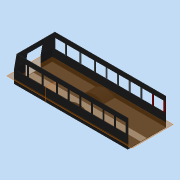
# Autodesk Inventor part: Pickle Interior
Saved by Autodesk Inventor 2018.2 (Build 222227000, 227)
## iProperties
Created: 2018-02-21
Part Number: Pickle Interior
Material: Generic
Document SubType Name: Modeling
Designer: owner
Density: 1 g/cm^3
Appearance: Default
Author: owner
Autodesk Inventor part; units mm, degrees
ref_plane "YZ Plane" through (0, 0, 0) normal (1, 0, 0) x (0, 1, 0)
ref_plane "XZ Plane" through (0, 0, 0) normal (0, 1, 0) x (-1, 0, 0)
ref_plane "XY Plane" through (0, 0, 0) normal (0, 0, 1) x (1, 0, 0)
sketch "Sketch1" plane through (0, 0, 0) normal (0, 1, 0) x (-1, 0, 0)
  line L0 (0, 0) -> (-6985, 0)
  line L1 (-6985, 0) -> (-6985, -2349.5)
  line L2 (-6985, -2349.5) -> (0, -2349.5)
  line L3 (0, -2349.5) -> (0, 0)
  dimension "d0" = 6985
  dimension "d1" = 2349.5
  constraints: 8 end point, 2 parallel, 1 horizontal, 1 perpendicular
  measures "d0" distance of L2.end L1.end
  measures "d1" distance of L1.end L0.end
extrude "Extrusion1" add sketch "Sketch1" along normal blind 25.4
sketch "Sketch2" plane through (0, 25.4, 0) normal (0, 1, 0) x (1, 0, 0)
  line L0 (0, 0) -> (6985, 0) projected
  line L1 (6985, 0) -> (6985, 2349.5) projected
  line L2 (6985, 2349.5) -> (0, 2349.5) projected
  line L3 (0, 2349.5) -> (0, 0) projected
  line L4 (6985, 25.4) -> (25.4, 25.4)
  line L5 (25.4, 25.4) -> (25.4, 2324.1)
  line L6 (25.4, 2324.1) -> (6985, 2324.1)
  dimension "d4" = 25.4
  constraints: 6 end point, 2 point on line
  measures "d4" distance between parallel lines of L0 L4
extrude "Extrusion2" add sketch "Sketch2" along normal blind 1644.65 contours L3 L2 L1 L6 L5 L4 L0
sketch "Sketch3" plane through (0, 0, 0) normal (0, 0, 1) x (1, 0, 0)
  line L0 (25.4, 25.4) -> (25.4, 742.95)
  line L1 (25.4, 742.95) -> (190.5, 742.95)
  line L2 (190.5, 742.95) -> (190.5, 1670.05)
  line L3 (25.4, 1670.05) -> (6985, 1670.05) projected
  line L4 (25.4, 742.95) -> (190.5, 1670.05)
  line L5 (190.5, 1670.05) -> (165.1, 1670.05)
  line L6 (165.1, 1670.05) -> (0, 742.95)
  line L7 (0, 0) -> (0, 1670.05) projected
  line L8 (0, 742.95) -> (0, 1670.05)
  line L9 (0, 1670.05) -> (165.1, 1670.05)
  line L10 (0, 742.95) -> (25.4, 742.95)
  dimension "d7" = 717.55
  dimension "d9" = 25.4
  constraints: 18 end point, 3 perpendicular, 3 point on line, 1 collinear, 1 parallel
  measures "d7" distance of L0.start L0.end
  measures "d9" distance of L2.end L5.end
extrude "Extrusion3" cut sketch "Sketch3" against normal up to surface (2349.5 mm away) contours L7 L9 L3 L6
extrude "Extrusion4" add sketch "Sketch3" against normal up to surface (2349.5 mm away) contours L10 L6 L3 L4
sketch "Sketch5" plane through (25.4, 25.4, -2324.1) normal (0, 0, 1) x (1, 0, 0)
  line L0 (6959.6, 0) -> (0, 0) projected
  line L1 (0, 0) -> (165.1, 0)
  line L2 (165.1, 0) -> (165.1, 749.3)
  line L3 (165.1, 749.3) -> (787.4, 749.3)
  line L4 (787.4, 749.3) -> (787.4, 1352.55)
  line L5 (787.4, 1352.55) -> (165.1, 1352.55)
  line L6 (165.1, 1352.55) -> (165.1, 749.3)
  line L7 (787.4, 1050.925) -> (876.3, 1050.925)
  line L8 (876.3, 749.3) -> (1676.4, 749.3)
  line L9 (1676.4, 749.3) -> (1676.4, 1352.55)
  line L10 (1676.4, 1352.55) -> (876.3, 1352.55)
  line L11 (876.3, 1352.55) -> (876.3, 749.3)
  line L12 (1676.4, 1050.925) -> (1765.3, 1050.925)
  line L13 (1676.4, 1050.925) -> (1765.3, 1050.925) construction
  line L14 (1765.3, 749.3) -> (2565.4, 749.3)
  line L15 (2565.4, 749.3) -> (2565.4, 1352.55)
  line L16 (2565.4, 1352.55) -> (1765.3, 1352.55)
  line L17 (1765.3, 1352.55) -> (1765.3, 749.3)
  line L18 (2565.4, 1050.925) -> (2654.3, 1050.925)
  line L19 (2654.3, 749.3) -> (3276.6, 749.3)
  line L20 (3276.6, 749.3) -> (3276.6, 1352.55)
  line L21 (3276.6, 1352.55) -> (2654.3, 1352.55)
  line L22 (2654.3, 1352.55) -> (2654.3, 749.3)
  line L23 (3276.6, 1050.925) -> (3365.5, 1050.925)
  line L24 (3365.5, 749.3) -> (3987.8, 749.3)
  line L25 (3987.8, 749.3) -> (3987.8, 1352.55)
  line L26 (3987.8, 1352.55) -> (3365.5, 1352.55)
  line L27 (3365.5, 1352.55) -> (3365.5, 749.3)
  line L28 (3987.8, 1050.925) -> (4076.7, 1050.925)
  line L29 (4699, 1050.925) -> (4787.9, 1050.925)
  line L30 (5410.2, 1050.925) -> (5499.1, 1050.925)
  line L31 (4076.7, 749.3) -> (4699, 749.3)
  line L32 (4699, 749.3) -> (4699, 1352.55)
  line L33 (4699, 1352.55) -> (4076.7, 1352.55)
  line L34 (4076.7, 1352.55) -> (4076.7, 749.3)
  line L35 (4787.9, 749.3) -> (5410.2, 749.3)
  line L36 (5410.2, 749.3) -> (5410.2, 1352.55)
  line L37 (5410.2, 1352.55) -> (4787.9, 1352.55)
  line L38 (4787.9, 1352.55) -> (4787.9, 749.3)
  line L39 (5499.1, 749.3) -> (6121.4, 749.3)
  line L40 (6121.4, 749.3) -> (6121.4, 1352.55)
  line L41 (6121.4, 1352.55) -> (5499.1, 1352.55)
  line L42 (5499.1, 1352.55) -> (5499.1, 749.3)
  line L43 (6121.4, 1050.925) -> (6216.65, 1050.925)
  line L44 (6216.65, 749.3) -> (6826.25, 749.3)
  line L45 (6826.25, 749.3) -> (6826.25, 1352.55)
  line L46 (6826.25, 1352.55) -> (6216.65, 1352.55)
  line L47 (6216.65, 1352.55) -> (6216.65, 749.3)
  line L48 (6826.25, 1050.925) -> (6921.5, 1050.925)
  line L49 (6921.5, 1050.925) -> (6921.5, 1326.0553)
  line L50 (6921.5, 1326.0553) -> (6959.6, 1326.0553)
  line L51 (6959.6, 0) -> (6959.6, 1644.65) projected
  point P0 (-25.4, -25.4)
  dimension "d16" = 165.1
  dimension "d17" = 749.3
  dimension "d18" = 622.3
  dimension "d19" = 603.25
  dimension "d20" = 88.9
  dimension "d21" = 800.1
  dimension "d22" = 88.9
  dimension "d24" = 800.1
  dimension "d25" = 88.9
  dimension "d26" = 622.3
  dimension "d27" = 88.9
  dimension "d28" = 622.3
  dimension "d29" = 88.9
  dimension "d30" = 622.3
  dimension "d31" = 88.9
  dimension "d32" = 622.3
  dimension "d33" = 88.9
  dimension "d35" = 622.3
  dimension "d36" = 95.25
  dimension "d37" = 609.6
  dimension "d38" = 95.25
  constraints: 100 end point, 18 parallel, 17 horizontal, 11 perpendicular, 7 midpoint, 7 point on line, 1 collinear, 1 vertical
  measures "d16" distance of L0.end L1.end
  measures "d17" distance of L1.end L2.end
  measures "d18" distance of L5.end L4.end
  measures "d19" distance of L4.end L3.end
  measures "d20" distance of L7.start L7.end
  measures "d21" distance of L10.end L9.end
  measures "d22" distance of L12.start L12.end
  measures "d24" distance of L16.end L15.end
  measures "d25" distance of L18.start L18.end
  measures "d26" distance of L21.end L20.end
  measures "d27" distance of L23.start L23.end
  measures "d28" distance of L26.end L25.end
  measures "d29" distance of L28.start L28.end
  measures "d30" distance of L28.end L29.start
  measures "d31" distance of L29.start L29.end
  measures "d32" distance of L29.end L30.start
  measures "d33" distance of L30.start L30.end
  measures "d35" distance of L41.end L40.end
  measures "d36" distance of L43.start L43.end
  measures "d37" distance of L46.end L45.end
  measures "d38" distance of L48.start L48.end
extrude "Extrusion6" cut sketch "Sketch5" against normal blind 25.4 contours L6 L5 L4 L3
extrude "Extrusion7" cut sketch "Sketch5" against normal blind 25.4 contours L11 L10 L9 L8
extrude "Extrusion8" cut sketch "Sketch5" against normal blind 25.4 contours L17 L16 L15 L14
extrude "Extrusion9" cut sketch "Sketch5" against normal blind 25.4 contours L22 L21 L20 L19
extrude "Extrusion10" cut sketch "Sketch5" against normal blind 25.4 contours L27 L26 L25 L24
extrude "Extrusion11" cut sketch "Sketch5" against normal blind 25.4 contours L32 L31 L34 L33
extrude "Extrusion12" cut sketch "Sketch5" against normal blind 25.4 contours L36 L35 L38 L37
extrude "Extrusion13" cut sketch "Sketch5" against normal blind 25.4 contours L40 L39 L42 L41
extrude "Extrusion14" cut sketch "Sketch5" against normal blind 25.4 contours L45 L44 L47 L46
sketch "Sketch6" plane through (25.4, 25.4, -2324.1) normal (0, 0, 1) x (1, 0, 0)
  line L0 (787.4, 1352.55) -> (787.4, 749.3) projected
  line L1 (876.3, 749.3) -> (876.3, 1352.55) projected
  line L2 (1676.4, 1352.55) -> (1676.4, 749.3) projected
  line L3 (1765.3, 749.3) -> (1765.3, 1352.55) projected
  line L4 (2565.4, 1352.55) -> (2565.4, 749.3) projected
  line L5 (2654.3, 749.3) -> (2654.3, 1352.55) projected
  line L6 (3276.6, 1352.55) -> (3276.6, 749.3) projected
  line L7 (3365.5, 749.3) -> (3365.5, 1352.55) projected
  line L8 (3987.8, 1352.55) -> (3987.8, 749.3) projected
  line L9 (4076.7, 749.3) -> (4076.7, 1352.55) projected
  line L10 (4699, 1352.55) -> (4699, 749.3) projected
  line L11 (4787.9, 749.3) -> (4787.9, 1352.55) projected
  line L12 (5410.2, 1352.55) -> (5410.2, 749.3) projected
  line L13 (5499.1, 749.3) -> (5499.1, 1352.55) projected
  line L14 (6121.4, 1352.55) -> (6121.4, 749.3) projected
  line L15 (6216.65, 749.3) -> (6216.65, 1352.55) projected
  line L16 (6826.25, 1352.55) -> (6826.25, 749.3) projected
  line L17 (6826.25, 1352.55) -> (6921.5, 1352.55)
  line L18 (6921.5, 1352.55) -> (6921.5, 749.3)
  line L19 (165.1, 1352.55) -> (165.1, 749.3) projected
  line L20 (787.4, 1352.55) -> (876.3, 1352.55)
  line L21 (876.3, 749.3) -> (787.4, 749.3)
  line L22 (1676.4, 1352.55) -> (1765.3, 1352.55)
  line L23 (1765.3, 749.3) -> (1676.4, 749.3)
  line L24 (2654.3, 749.3) -> (2565.4, 749.3)
  line L25 (2565.4, 1352.55) -> (2654.3, 1352.55)
  line L26 (3276.6, 1352.55) -> (3365.5, 1352.55)
  line L27 (3365.5, 749.3) -> (3276.6, 749.3)
  line L28 (4076.7, 749.3) -> (3987.8, 749.3)
  line L29 (3987.8, 1352.55) -> (4076.7, 1352.55)
  line L30 (4699, 1352.55) -> (4787.9, 1352.55)
  line L31 (4787.9, 749.3) -> (4699, 749.3)
  line L32 (5499.1, 749.3) -> (5410.2, 749.3)
  line L33 (5410.2, 1352.55) -> (5499.1, 1352.55)
  line L34 (6121.4, 1352.55) -> (6216.65, 1352.55)
  line L35 (6921.5, 749.3) -> (6826.25, 749.3)
  line L36 (6216.65, 749.3) -> (6121.4, 749.3)
  point P0 (-25.4, -25.4)
  dimension "d57" = 95.25
  constraints: 68 end point, 18 perpendicular, 3 point on line, 1 horizontal
  measures "d57" distance of L16.start L17.end
extrude "Extrusion15" add sketch "Sketch6" along normal blind 6.35 contours L20 L1 L21 L0
extrude "Extrusion16" add sketch "Sketch6" along normal blind 6.35 contours L22 L3 L23 L2
extrude "Extrusion17" add sketch "Sketch6" along normal blind 6.35 contours L25 L5 L24 L4
extrude "Extrusion18" add sketch "Sketch6" along normal blind 6.35 contours L26 L7 L27 L6
extrude "Extrusion19" add sketch "Sketch6" along normal blind 6.35 contours L29 L9 L28 L8
extrude "Extrusion20" add sketch "Sketch6" along normal blind 6.35 contours L30 L11 L31 L10
extrude "Extrusion21" add sketch "Sketch6" along normal blind 6.35 contours L33 L13 L32 L12
extrude "Extrusion22" add sketch "Sketch6" along normal blind 6.35 contours L34 L15 L36 L14
extrude "Extrusion23" add sketch "Sketch6" along normal blind 6.35 contours L17 L18 L35 L16
sketch "Sketch7" plane through (6985, 25.4, -25.4) normal (0, 0, -1) x (-1, 0, 0)
  line L0 (133.35, 1352.55) -> (742.95, 1352.55) projected
  line L1 (742.95, 749.3) -> (133.35, 749.3) projected
  line L2 (838.2, 749.3) -> (838.2, 1352.55) projected
  line L3 (838.2, 1352.55) -> (1460.5, 1352.55) projected
  line L4 (1460.5, 1352.55) -> (1460.5, 749.3) projected
  line L5 (1460.5, 749.3) -> (838.2, 749.3) projected
  line L6 (1549.4, 749.3) -> (1549.4, 1352.55) projected
  line L7 (1549.4, 1352.55) -> (2171.7, 1352.55) projected
  line L8 (2171.7, 1352.55) -> (2171.7, 749.3) projected
  line L9 (2171.7, 749.3) -> (1549.4, 749.3) projected
  line L10 (2260.6, 749.3) -> (2260.6, 1352.55) projected
  line L11 (2260.6, 1352.55) -> (2882.9, 1352.55) projected
  line L12 (2882.9, 1352.55) -> (2882.9, 749.3) projected
  line L13 (2882.9, 749.3) -> (2260.6, 749.3) projected
  line L14 (2971.8, 749.3) -> (2971.8, 1352.55) projected
  line L15 (2971.8, 1352.55) -> (3594.1, 1352.55) projected
  line L16 (3594.1, 1352.55) -> (3594.1, 749.3) projected
  line L17 (3594.1, 749.3) -> (2971.8, 749.3) projected
  line L18 (3683, 749.3) -> (3683, 1352.55) projected
  line L19 (3683, 1352.55) -> (4305.3, 1352.55) projected
  line L20 (4305.3, 1352.55) -> (4305.3, 749.3) projected
  line L21 (4305.3, 749.3) -> (3683, 749.3) projected
  line L22 (4400.55, 1352.55) -> (5187.95, 1352.55)
  line L23 (5187.95, 749.3) -> (4400.55, 749.3)
  line L24 (5283.2, 749.3) -> (5283.2, 1352.55) projected
  line L25 (5283.2, 1352.55) -> (6083.3, 1352.55) projected
  line L26 (6083.3, 1352.55) -> (6083.3, 749.3) projected
  line L27 (6083.3, 749.3) -> (5283.2, 749.3) projected
  line L28 (6172.2, 749.3) -> (6172.2, 1352.55) projected
  line L29 (6172.2, 1352.55) -> (6794.5, 1352.55) projected
  line L30 (6794.5, 1352.55) -> (6794.5, 749.3) projected
  line L31 (6794.5, 749.3) -> (6172.2, 749.3) projected
  line L32 (6985, 717.55) -> (6819.9, 1644.65) projected
  line L33 (0, 1644.65) -> (6819.9, 1644.65) projected
  line L34 (0, -25.4) -> (0, 1644.65) projected
  line L35 (0, -25.4) -> (6985, -25.4) projected
  line L36 (6985, -25.4) -> (6985, 717.55) projected
  line L37 (127, 1352.55) -> (127, 749.3)
  line L38 (127, 749.3) -> (749.3, 749.3)
  line L39 (749.3, 749.3) -> (749.3, 1352.55)
  line L40 (127, 1352.55) -> (749.3, 1352.55)
  line L41 (4400.55, 1352.55) -> (4400.55, 749.3)
  line L42 (5187.95, 749.3) -> (5187.95, 1352.55)
  constraints: 16 end point, 2 vertical, 1 perpendicular
extrude "Extrusion24" cut sketch "Sketch7" against normal blind 25.4 contours L0 L40 L39 L38 L1 L37
extrude "Extrusion25" cut sketch "Sketch7" against normal blind 25.4 contours L2 L3 L4 L5
extrude "Extrusion26" cut sketch "Sketch7" against normal blind 25.4 contours L6 L7 L8 L9
extrude "Extrusion27" cut sketch "Sketch7" against normal blind 25.4 contours L10 L11 L12 L13
extrude "Extrusion28" cut sketch "Sketch7" against normal blind 25.4 contours L14 L15 L16 L17
extrude "Extrusion29" cut sketch "Sketch7" against normal blind 25.4 contours L18 L19 L20 L21
extrude "Extrusion30" cut sketch "Sketch7" against normal blind 25.4 contours L22 L42 L23 L41
extrude "Extrusion31" cut sketch "Sketch7" against normal blind 25.4 contours L24 L25 L26 L27
extrude "Extrusion32" cut sketch "Sketch7" against normal blind 25.4 contours L28 L29 L30 L31
sketch "Sketch8" plane through (6985, 25.4, -25.4) normal (0, 0, -1) x (-1, 0, 0)
  line L0 (6794.5, 1352.55) -> (6172.2, 1352.55) projected
  line L1 (6794.5, 1352.55) -> (6794.5, 749.3) projected
  line L2 (6794.5, 1352.55) -> (6794.5, 749.3)
  line L3 (749.3, 749.3) -> (127, 749.3) projected
  line L4 (749.3, 1352.55) -> (749.3, 749.3) projected
  line L5 (838.2, 749.3) -> (838.2, 1352.55) projected
  line L6 (1460.5, 1352.55) -> (1460.5, 749.3) projected
  line L7 (1549.4, 749.3) -> (1549.4, 1352.55) projected
  line L8 (6794.5, 749.3) -> (6172.2, 749.3) projected
  line L9 (6172.2, 749.3) -> (6172.2, 1352.55) projected
  line L10 (6172.2, 1352.55) -> (6794.5, 1352.55) projected
  line L11 (6794.5, 1352.55) -> (6794.5, 749.3) projected
  line L12 (6083.3, 749.3) -> (5283.2, 749.3) projected
  line L13 (5283.2, 749.3) -> (5283.2, 1352.55) projected
  line L14 (5283.2, 1352.55) -> (6083.3, 1352.55) projected
  line L15 (6083.3, 1352.55) -> (6083.3, 749.3) projected
  line L16 (5187.95, 1352.55) -> (5187.95, 749.3) projected
  line L17 (5187.95, 749.3) -> (4400.55, 749.3) projected
  line L18 (4400.55, 749.3) -> (4400.55, 1352.55) projected
  line L19 (4400.55, 1352.55) -> (5187.95, 1352.55) projected
  line L20 (4305.3, 749.3) -> (3683, 749.3) projected
  line L21 (3683, 749.3) -> (3683, 1352.55) projected
  line L22 (3683, 1352.55) -> (4305.3, 1352.55) projected
  line L23 (4305.3, 1352.55) -> (4305.3, 749.3) projected
  line L24 (3594.1, 749.3) -> (2971.8, 749.3) projected
  line L25 (2971.8, 749.3) -> (2971.8, 1352.55) projected
  line L26 (2971.8, 1352.55) -> (3594.1, 1352.55) projected
  line L27 (3594.1, 1352.55) -> (3594.1, 749.3) projected
  line L28 (2882.9, 749.3) -> (2260.6, 749.3) projected
  line L29 (2260.6, 749.3) -> (2260.6, 1352.55) projected
  line L30 (2260.6, 1352.55) -> (2882.9, 1352.55) projected
  line L31 (2882.9, 1352.55) -> (2882.9, 749.3) projected
  line L32 (2171.7, 749.3) -> (1549.4, 749.3) projected
  line L33 (1549.4, 749.3) -> (1549.4, 1352.55) projected
  line L34 (1549.4, 1352.55) -> (2171.7, 1352.55) projected
  line L35 (2171.7, 1352.55) -> (2171.7, 749.3) projected
  line L36 (1460.5, 749.3) -> (838.2, 749.3) projected
  line L37 (838.2, 749.3) -> (838.2, 1352.55) projected
  line L38 (838.2, 1352.55) -> (1460.5, 1352.55) projected
  line L39 (1460.5, 1352.55) -> (1460.5, 749.3) projected
  line L40 (749.3, 749.3) -> (127, 749.3) projected
  line L41 (127, 749.3) -> (127, 1352.55) projected
  line L42 (127, 1352.55) -> (749.3, 1352.55) projected
  line L43 (749.3, 1352.55) -> (749.3, 749.3) projected
  line L44 (6959.6, 717.55) -> (6794.5, 1644.65) projected
  line L45 (0, 1644.65) -> (6794.5, 1644.65) projected
  line L46 (0, 0) -> (0, 1644.65) projected
  line L47 (6959.6, 0) -> (0, 0) projected
  line L48 (6959.6, 0) -> (6959.6, 717.55) projected
  line L49 (3594.1, 1352.55) -> (3683, 1352.55)
  line L50 (4305.3, 1352.55) -> (4400.55, 1352.55)
  line L51 (6172.2, 749.3) -> (6083.3, 749.3)
  line L52 (5283.2, 749.3) -> (5187.95, 749.3)
  line L53 (5187.95, 1352.55) -> (5283.2, 1352.55)
  line L54 (6083.3, 1352.55) -> (6172.2, 1352.55)
  line L55 (4400.55, 749.3) -> (4305.3, 749.3)
  line L56 (3683, 749.3) -> (3594.1, 749.3)
  line L57 (2971.8, 749.3) -> (2882.9, 749.3)
  line L58 (2882.9, 1352.55) -> (2971.8, 1352.55)
  line L59 (2171.7, 1352.55) -> (2260.6, 1352.55)
  line L60 (2260.6, 749.3) -> (2171.7, 749.3)
  line L61 (1549.4, 749.3) -> (1460.5, 749.3)
  line L62 (838.2, 749.3) -> (749.3, 749.3)
  line L63 (749.3, 1352.55) -> (838.2, 1352.55)
  line L64 (1460.5, 1352.55) -> (1549.4, 1352.55)
  line L65 (127, 749.3) -> (38.1, 749.3)
  line L66 (38.1, 749.3) -> (38.1, 1352.55)
  line L67 (38.1, 1352.55) -> (127, 1352.55)
  line L68 (127, 1352.55) -> (127, 749.3)
  point P0 (6985, -25.4)
  dimension "d100" = 88.9
  constraints: 72 end point, 16 collinear, 9 perpendicular, 3 point on line, 2 parallel, 1 horizontal
  measures "d100" distance of L66.end L67.end
extrude "Extrusion33" add sketch "Sketch8" along normal blind 6.35 contours L5 L62 L4 L63
extrude "Extrusion34" add sketch "Sketch8" along normal blind 6.35 contours L41 L65 L66 L67
extrude "Extrusion35" add sketch "Sketch8" along normal blind 6.35 contours L7 L61 L6 L64
extrude "Extrusion36" add sketch "Sketch8" along normal blind 6.35 contours L29 L60 L35 L59
extrude "Extrusion37" add sketch "Sketch8" along normal blind 6.35 contours L25 L57 L31 L58
extrude "Extrusion38" add sketch "Sketch8" along normal blind 6.35 contours L21 L56 L27 L49
extrude "Extrusion39" add sketch "Sketch8" along normal blind 6.35 contours L18 L55 L23 L50
extrude "Extrusion40" add sketch "Sketch8" along normal blind 6.35 contours L13 L52 L16 L53
extrude "Extrusion41" add sketch "Sketch8" along normal blind 6.35 contours L9 L51 L15 L54
sketch "Sketch9" plane through (6985, 25.4, -25.4) normal (0, 0, -1) x (-1, 0, 0)
  line L0 (6959.6, 0) -> (0, 0) projected
  line L1 (6959.6, 0) -> (4305.3, 0)
  line L2 (6959.6, 0) -> (9613.9, 0) construction
  line L3 (4305.3, 0) -> (3124.2, 0)
  arc A0 (4305.3, 0) -> (3124.2, 0) centre (3714.75, -756.543) ccw
  point P0 (6985, -25.4)
  dimension "d117" = 2654.3
  dimension "d118" = 180
  dimension "d119" = 1181.1
  constraints: 6 end point, 2 collinear, 2 point on circle, 1 centre point, 1 horizontal, 1 point on line
  measures "d117" distance of L0.start L1.end
  measures "d118" angle of L1 L2
  measures "d119" distance of L1.end L3.end
extrude "Extrusion42" add sketch "Sketch9" along normal blind 660.4
sketch "Sketch10" plane through (25.4, 25.4, -2324.1) normal (0, 0, 1) x (1, 0, 0)
  line L0 (6959.6, 0) -> (0, 0) projected
  line L1 (0, 0) -> (2654.3, 0)
  line L2 (2654.3, 0) -> (3835.4, 0)
  arc A0 (3835.4, 0) -> (2654.3, 0) centre (3244.85, -756.543) ccw
  point P0 (-25.4, -25.4)
  dimension "d123" = 2654.3
  dimension "d124" = 1181.1
  constraints: 4 end point, 2 point on circle, 2 point on line, 1 centre point
  measures "d123" distance of L0.end L1.end
  measures "d124" distance of L1.end L2.end
extrude "Extrusion43" add sketch "Sketch10" along normal blind 660.4
sketch "Sketch11" plane through (0, 25.4, 0) normal (0, 1, 0) x (1, 0, 0)
  line L0 (6985, 25.4) -> (6985, 793.75)
  line L1 (6985, 25.4) -> (6985, 2324.1) projected
  line L2 (25.4, 2324.1) -> (25.4, 25.4) projected
  line L3 (6985, 793.75) -> (25.4, 793.75)
  line L4 (25.4, 793.75) -> (25.4, 1168.4)
  line L5 (25.4, 1168.4) -> (6985, 1168.4)
  line L6 (6985, 1168.4) -> (6985, 793.75)
  line L7 (6984.9746, 1168.3746) -> (25.4254, 1168.3746)
  line L8 (25.4254, 1168.3746) -> (25.4254, 793.7754)
  line L9 (25.4254, 793.7754) -> (6984.9746, 793.7754)
  line L10 (6984.9746, 793.7754) -> (6984.9746, 1168.3746)
  point P0 (0, 0)
  dimension "d128" = 768.35
  dimension "d129" = 374.65
  dimension "d130" = 0.0254
  constraints: 18 end point, 4 parallel, 2 perpendicular, 2 point on line, 1 horizontal, 3 other
  measures "d128" distance of L0.start L0.end
  measures "d129" distance of L3.end L4.end
  measures "d130" distance between parallel lines of L5 L7
extrude "Extrusion44" cut sketch "Sketch11" against normal blind 0.0254
sketch "Sketch12" plane through (0, 0, -2349.5) normal (-1, 0, 0) x (0, 0, 1)
  line L0 (2324.1, 25.4) -> (1555.75, 25.4) projected
  line L1 (2324.1, 25.4) -> (1647.825, 25.4)
  line L2 (1647.825, 25.4) -> (1647.825, 1314.45)
  line L3 (1663.7, 228.6) -> (1663.7, 25.4) projected
  line L4 (1647.825, 25.4) -> (2936.875, 25.4) construction
  line L5 (1647.825, 1314.45) -> (701.675, 1314.45)
  line L6 (701.675, 1314.45) -> (701.675, 25.4)
  line L7 (701.675, 25.4) -> (1647.825, 25.4)
  point P0 (2349.5, 0)
  dimension "d133" = 676.275
  dimension "d134" = 1289.05
  dimension "d135" = 90
  dimension "d136" = 946.15
  constraints: 12 end point, 4 perpendicular, 1 horizontal, 1 parallel, 1 point on line
  measures "d133" distance of L0.start L1.end
  measures "d134" distance of L1.end L2.end
  measures "d135" angle of L4 L2
  measures "d136" distance of L2.end L5.end
extrude "Extrusion45" cut sketch "Sketch12" against normal blind 338.1629
ref_plane "Work Plane1" through (1949.45, 25.4, -25.4) normal (1, 0, 0) x (0, 0, -1)
sketch "Sketch13" plane through (1949.45, 25.4, -25.4) normal (1, 0, 0) x (0, 0, -1)
  line L0 (0, 0) -> (406.4, 0)
  line L1 (0, 228.6) -> (0, 0)
  line L2 (0, 228.6) -> (406.4, 0)
  point P0 (-25.4, -25.4)
  constraints: 6 end point, 1 horizontal
extrude "Extrusion46" add sketch "Sketch13" along normal blind 212.725
ref_plane "Work Plane2" through (0, 288.925, 0) normal (0, 1, 0) x (1, 0, 0)
sketch "Sketch14" plane through (0, 288.925, 0) normal (0, 1, 0) x (1, 0, 0)
  line L0 (6985, 0) -> (6985, 2349.5) projected
  line L1 (158.75, 25.4) -> (6985, 25.4)
  line L2 (6985, 25.4) -> (6985, 53.975)
  line L3 (6985, 53.975) -> (158.75, 53.975)
  line L4 (158.75, 53.975) -> (158.75, 25.4)
  point P0 (0, 0)
  dimension "d145" = 28.575
  constraints: 8 end point, 2 parallel, 1 horizontal, 1 perpendicular, 1 point on line
  measures "d145" distance of L2.end L1.end
extrude "Extrusion47" add sketch "Sketch14" against normal blind 6.35
sketch "Sketch15" plane through (0, 288.925, 0) normal (0, 1, 0) x (1, 0, 0)
  line L0 (158.75, 53.975) -> (6985, 53.975) projected
  line L1 (158.75, 53.975) -> (158.75, 2524.0506)
  line L2 (6985, 2349.5) -> (0, 2349.5) projected
  line L3 (2679.7, 2324.1) -> (25.4, 2324.1) projected
  line L4 (158.75, 2324.1) -> (6985, 2324.1)
  line L5 (6985, 2324.1) -> (6985, 2295.525)
  line L6 (6985, 2295.525) -> (158.75, 2295.525)
  line L7 (158.75, 2295.525) -> (158.75, 2324.1)
  point P0 (0, 0)
  dimension "d148" = 28.575
  constraints: 10 end point, 2 parallel, 2 perpendicular, 2 point on line, 1 horizontal
  measures "d148" distance of L4.end L5.end
extrude "Extrusion48" add sketch "Sketch15" against normal blind 6.35
body "Solid1"
